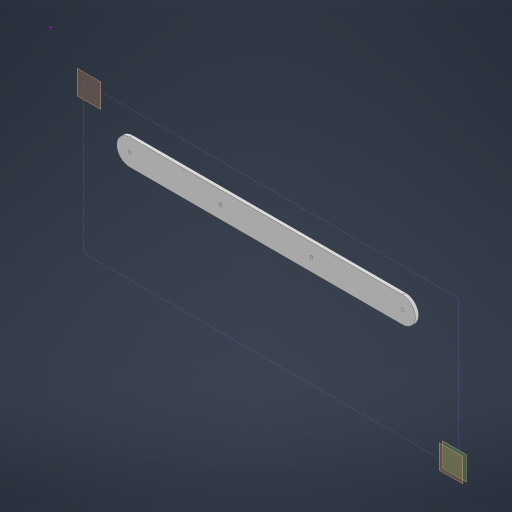
# Autodesk Inventor part: foot3
Saved by Autodesk Inventor 2024.2 (Build 282272000, 272)
## iProperties
Created: 2024-06-20
Part Number: foot3
Material: Generic
Document SubType Name: Modeling
Designer: Moe
Density: 1 g/cm^3
Appearance: Default
Author: Moe
Autodesk Inventor part; units mm, degrees
ref_plane "YZ Plane" through (0, 0, 0) normal (1, 0, 0) x (0, 1, 0)
ref_plane "XZ Plane" through (0, 0, 0) normal (0, 1, 0) x (-1, 0, 0)
ref_plane "XY Plane" through (0, 0, 0) normal (0, 0, 1) x (1, 0, 0)
ref_plane "Work Plane2" through (35.545, -31.609, 1.6) normal (0, 0, 1) x (1, 0, 0)
sketch "Sketch2" plane through (35.545, -31.609, 1.6) normal (0, 0, 1) x (1, 0, 0)
  line L0 (-4.7778, 3.1171) -> (341.5466, 3.1925) construction
  line L1 (341.5466, 3.1925) -> (341.5765, -133.848) construction
  line L2 (341.5765, -133.848) -> (-4.7479, -133.9235) construction
  line L3 (-4.7479, -133.9235) -> (-4.7778, 3.1171) construction
  point P0 (-35.545, 31.609)
  constraints: 2 other
ref_plane "Work Plane1" through (371.545, -162.609, 0) normal (0, 0, -1) x (-1, 0, 0)
ref_plane "Work Plane3" through (371.545, -162.609, 0) normal (0, 0, 1) x (1, 0, 0)
ref_plane "Work Plane4" through (371.545, -162.609, 3) normal (0, 0, 1) x (1, 0, 0)
sketch "Sketch11" plane through (371.545, -162.609, 3) normal (0, 0, 1) x (1, 0, 0)
  line L0 (-41.979, 113.527) -> (-294.039, 113.527) projected
  arc A0 (-294.039, 113.527) -> (-294.039, 93.527) centre (-294.039, 103.527) ccw projected
  line L1 (-294.039, 93.527) -> (-41.979, 93.527) projected
  arc A1 (-41.979, 93.527) -> (-41.979, 113.527) centre (-41.979, 103.527) ccw projected
  circle A2 centre (-41.979, 103.44) radius 1.1 projected
  circle A3 centre (-125.979, 103.44) radius 1.1 projected
  circle A4 centre (-210.039, 103.527) radius 1.1 projected
  circle A5 centre (-294.039, 103.527) radius 1.1 projected
  line L2 (-294.039, 115.527) -> (-41.979, 115.527)
  line L3 (-29.979, 103.527) -> (-29.979, 103.527)
  line L4 (-41.979, 91.527) -> (-294.039, 91.527)
  line L5 (-306.039, 103.527) -> (-306.039, 103.527)
  arc A6 (-41.979, 91.527) -> (-29.979, 103.527) centre (-41.979, 103.527) ccw
  arc A7 (-29.979, 103.527) -> (-41.979, 115.527) centre (-41.979, 103.527) ccw
  arc A8 (-306.039, 103.527) -> (-294.039, 91.527) centre (-294.039, 103.527) ccw
  arc A9 (-294.039, 115.527) -> (-306.039, 103.527) centre (-294.039, 103.527) ccw
  point P0 (-371.545, 162.609)
  point P1 (-31.979, 103.527)
  point P2 (-304.039, 103.527)
  point P3 (-29.979, 103.527)
  point P4 (-29.979, 103.527)
  dimension "d109" = 12
  dimension "d110" = 12
  dimension "d111" = 12
  dimension "d112" = 12
  dimension "d113" = 12
  constraints: 10 point on circle, 8 end point, 8 tangent, 4 centre point, 3 equal radius, 2 parallel, 1 horizontal, 1 midpoint, 1 perpendicular
  measures "d109" distance from line of A0.centre L5
  measures "d110" distance from line of A0.centre L2
  measures "d111" distance from line of L4 A0.centre
  measures "d112" distance of point (-29.979, 103.527) A1.centre
  measures "d113" radius of A6
extrude "Extrusion7" add sketch "Sketch11" along normal blind 3 contours A1 L1 A0 L0 | L2 A7 A6 L4 A8 A9
body "Solid2"
